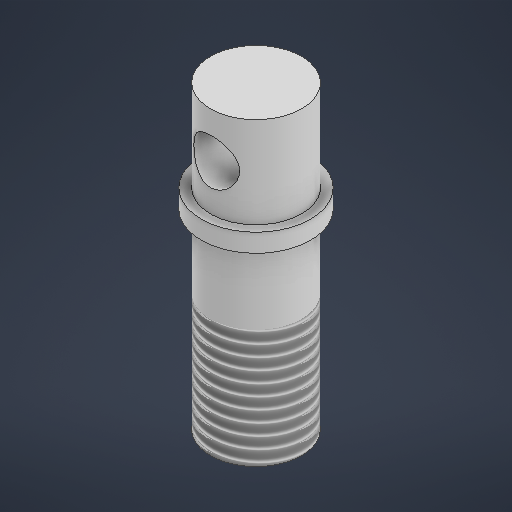
# Autodesk Inventor part: Pieza4
Saved by Autodesk Inventor 2026.1 (Build 301233000, 233)
## iProperties
Created: 2025-09-19
Part Number: Pieza4
Material: Genérico
Document SubType Name: Modeling
Designer: Usuario
Density: 1 g/cm^3
Appearance: Valor por defecto
Author: Usuario
Autodesk Inventor part; units mm, degrees
ref_plane "YZ Plane" through (0, 0, 0) normal (1, 0, 0) x (0, 1, 0)
ref_plane "XZ Plane" through (0, 0, 0) normal (0, 1, 0) x (-1, 0, 0)
sketch "Boceto1" plane through (0, 0, 0) normal (0, 1, 0) x (-1, 0, 0)
  circle A0 centre (0, 0) radius 5
  dimension "d0" = 10
  constraints: 1 centre point, 1 coincident
  measures "d0" diameter of A0
extrude "Extrusión1" add sketch "Boceto1" along normal blind 21
thread "Rosca1" size "M9x1.25" class "6g" standard "ANSI Metric M Profile" length 13
sketch "Boceto2" plane through (0, 21, 0) normal (0, 1, 0) x (1, 0, 0)
  circle A0 centre (0, 0) radius 6
  dimension "d5" = 12
  constraints: 1 centre point, 1 coincident
  measures "d5" diameter of A0
extrude "Extrusión2" add sketch "Boceto2" along normal blind 2
sketch "Boceto3" plane through (0, 23, 0) normal (0, 1, 0) x (1, 0, 0)
  circle A0 centre (0, 0) radius 5
  dimension "d8" = 10
  constraints: 1 centre point, 1 coincident
  measures "d8" diameter of A0
extrude "Extrusión3" add sketch "Boceto3" along normal blind 10
ref_plane "Plano de trabajo1" through (0, 23, 5) normal (0, 0, 1) x (1, 0, 0)
sketch "Boceto4" plane through (0, 23, 5) normal (0, 0, 1) x (1, 0, 0)
  line L0 (5, 10) -> (-5, 10) projected
  line L1 (-5, 10) -> (5.0514, 0) construction
  line L2 (6, 0) -> (-6, 0) projected
  line L3 (5, 0) -> (5, 10) projected
  line L4 (5, 10) -> (-4.9489, 0) construction
  circle A0 centre (0.0256, 5) radius 2.5
  point P0 (0, -23)
  dimension "d11" = 5
  constraints: 4 end point, 2 point on line, 1 centre point, 1 midpoint, 1 perpendicular
  measures "d11" diameter of A0
extrude "Extrusión4" cut sketch "Boceto4" against normal through all
